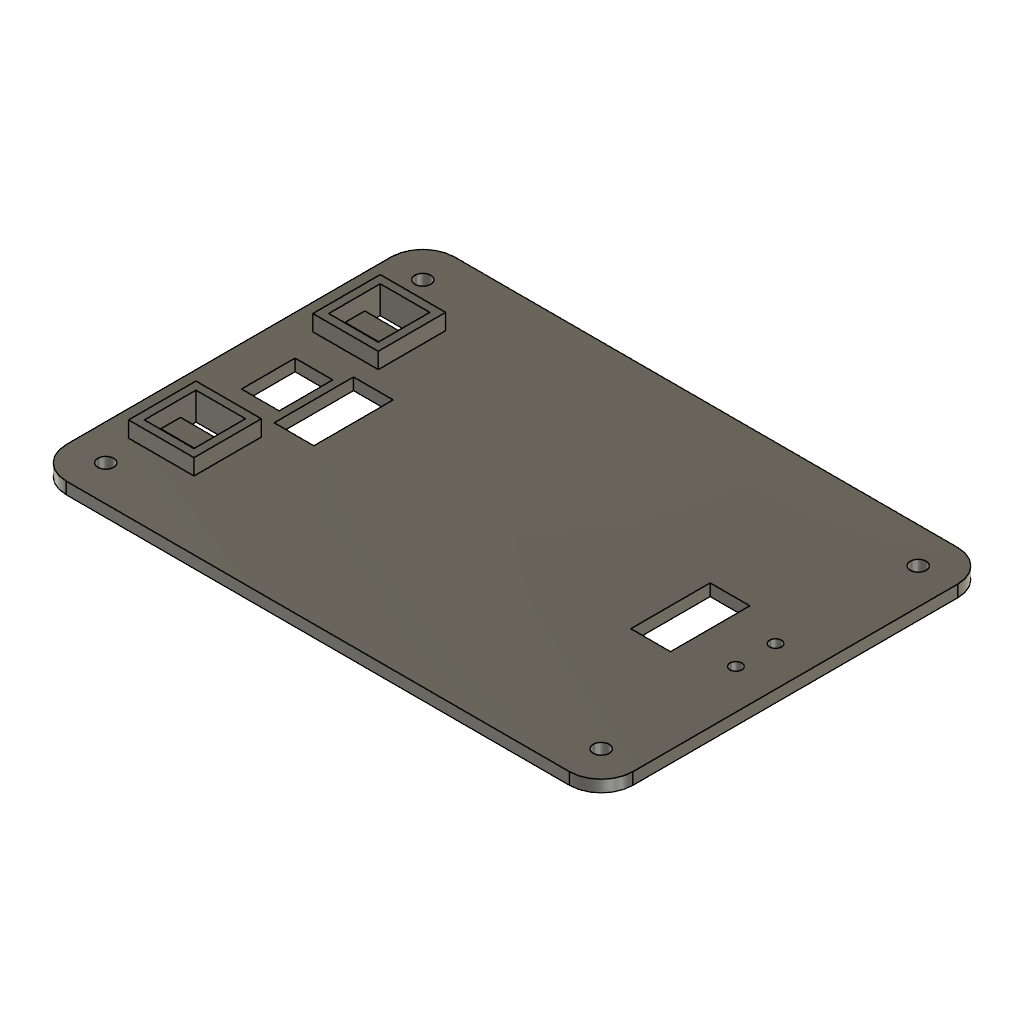
Tapa de la PCB (Autodesk Fusion 360 design; units mm, degrees)
Autodesk Fusion 360 part; units mm, degrees
sketch "Boceto1" plane through (0, 0, 0) normal (0, 0, 1) x (1, 0, 0)
  line L0 (71.5, 0) -> (-71.5, 0)
  line L1 (0, -49) -> (0, 49)
  line L2 (-71.5, 49) -> (71.5, 49)
  line L3 (71.5, 49) -> (71.5, -49)
  line L4 (71.5, -49) -> (-71.5, -49)
  line L5 (-71.5, -49) -> (-71.5, 49)
  line L6 (-71.5, 49) -> (71.5, -49) construction
  line L7 (71.5, 49) -> (-71.5, -49) construction
  dimension "d1" = 143
  dimension "d2" = 98
  constraint midpoint L0 origin
  constraint horizontal L0
  constraint midpoint L1 origin
  constraint perpendicular L0 L1
  constraint horizontal L2
  constraint perpendicular L2 L3
  constraint parallel L2 L4
  constraint parallel L3 L5
  constraint coincident L6 origin
  constraint coincident L7 origin
  measures "d1" distance of L0.start L0.end
  measures "d2" distance of L1.start L1.end
extrude "Extruir1" add sketch "Boceto1" along normal blind 3
sketch "Boceto2" plane through (0, 0, 3) normal (0, 0, 1) x (-1, 0, 0)
  line L0 (71.5, 49) -> (-71.5, 49)
  line L1 (-71.5, 49) -> (-71.5, -49)
  line L2 (-71.5, -49) -> (71.5, -49)
  line L3 (71.5, -49) -> (71.5, 49)
  line L4 (71.5, -49) -> (62.5, -49)
  line L5 (62.5, -49) -> (62.5, -40)
  line L6 (71.5, 49) -> (62.5, 49)
  line L7 (62.5, 49) -> (62.5, 40)
  line L8 (-71.5, 49) -> (-71.5, 40)
  line L9 (-71.5, 40) -> (-62.5, 40)
  line L10 (-71.5, -49) -> (-62.5, -49)
  line L11 (-62.5, -49) -> (-62.5, -40)
  circle A0 centre (62.5, -40) radius 2
  circle A1 centre (62.5, 40) radius 2
  circle A2 centre (-62.5, -40) radius 2
  circle A3 centre (-62.5, 40) radius 2
  dimension "d7" = 9
  dimension "d8" = 9
  dimension "d9" = 9
  dimension "d10" = 9
  dimension "d11" = 9
  dimension "d12" = 9
  dimension "d13" = 9
  dimension "d14" = 9
  dimension "d15" = 4
  dimension "d16" = 4
  dimension "d17" = 4
  dimension "d18" = 4
  constraint coincident L2.end L3.start
  constraint perpendicular L3 L4
  constraint perpendicular L2 L5
  constraint coincident L0.start L3.end
  constraint perpendicular L3 L6
  constraint perpendicular L6 L7
  constraint coincident L0.end L1.start
  constraint perpendicular L0 L8
  constraint perpendicular L1 L9
  constraint coincident L1.end L2.start
  constraint perpendicular L1 L10
  constraint perpendicular L2 L11
  constraint coincident L5.end A0.centre
  constraint coincident L7.end A1.centre
  constraint coincident L11.end A2.centre
  constraint coincident L9.end A3.centre
  measures "d7" distance of L2.end L4.end
  measures "d8" distance of L4.end L5.end
  measures "d9" distance of L0.start L6.end
  measures "d10" distance of L6.end L7.end
  measures "d11" distance of L0.end L8.end
  measures "d12" distance of L8.end L9.end
  measures "d13" distance of L1.end L10.end
  measures "d14" distance of L10.end L11.end
  measures "d15" diameter of A0
  measures "d16" diameter of A1
  measures "d17" diameter of A2
  measures "d18" diameter of A3
extrude "Extruir2" cut sketch "Boceto2" against normal blind 3 contours A0 | A1 | A2 | A3
fillet "Empalme2" radius 8 4 edges at (-71.5, -49, 1.5) (-71.5, 49, 1.5) (71.5, -49, 1.5) (71.5, 49, 1.5)
sketch "Boceto3" plane through (0, 0, 3) normal (0, 0, 1) x (-1, 0, 0)
  circle A0 centre (62.5, 40) radius 2
  circle A1 centre (-62.5, -40) radius 2
  circle A2 centre (62.5, -40) radius 2
  circle A3 centre (-62.5, 40) radius 2
  arc A4 (-71.5, -41) -> (-63.5, -49) centre (-63.5, -41) ccw
  line L0 (-63.5, -49) -> (63.5, -49)
  arc A5 (63.5, -49) -> (71.5, -41) centre (63.5, -41) ccw
  line L1 (71.5, -41) -> (71.5, 41)
  arc A6 (71.5, 41) -> (63.5, 49) centre (63.5, 41) ccw
  line L2 (63.5, 49) -> (-63.5, 49)
  arc A7 (-63.5, 49) -> (-71.5, 41) centre (-63.5, 41) ccw
  line L3 (-71.5, 41) -> (-71.5, -41)
  line L4 (-40, 0) -> (40, 0)
  line L5 (40, 10) -> (40, -10)
  line L6 (-40, 10) -> (-40, -10)
  line L7 (40, -10) -> (50, -10)
  line L8 (50, -10) -> (50, 10)
  line L9 (50, 10) -> (40, 10)
  line L10 (40, 10) -> (40, -10)
  line L11 (-40, -10) -> (-50, -10)
  line L12 (-50, -10) -> (-50, 10)
  line L13 (-50, 10) -> (-40, 10)
  line L14 (-40, 10) -> (-40, -10)
  dimension "d23" = 80
  dimension "d24" = 20
  dimension "d25" = 20
  dimension "d26" = 10
  dimension "d27" = 20
  dimension "d28" = 10
  dimension "d29" = 20
  constraint midpoint L4 origin
  constraint horizontal L4
  constraint midpoint L4.end L5
  constraint perpendicular L4 L5
  constraint midpoint L4.start L6
  constraint perpendicular L4 L6
  constraint horizontal L7
  constraint vertical L8
  constraint horizontal L9
  constraint vertical L10
  constraint horizontal L11
  constraint vertical L12
  constraint horizontal L13
  constraint vertical L14
  measures "d23" distance of L4.start L4.end
  measures "d24" distance of L5.start L5.end
  measures "d25" distance of L6.start L6.end
  measures "d26" distance of L5.end L7.end
  measures "d27" distance of L5.end L5.start
  measures "d28" distance of L6.end L11.end
  measures "d29" distance of L6.end L6.start
extrude "Extruir3" cut sketch "Boceto3" against normal blind 3 contours L5 L7 L8 L9 L10 | L6 L11 L12 L13 L14
sketch "Boceto4" plane through (0, 0, 3) normal (0, 0, 1) x (-1, 0, 0)
  line L0 (50, -10) -> (40, -10)
  line L1 (40, -10) -> (40, 10)
  line L2 (40, 10) -> (50, 10)
  line L3 (50, 10) -> (50, -10)
  line L4 (-50, -10) -> (-50, 10)
  line L5 (-50, 10) -> (-40, 10)
  line L6 (-40, 10) -> (-40, -10)
  line L7 (-40, -10) -> (-50, -10)
  circle A0 centre (62.5, 40) radius 2
  circle A1 centre (-62.5, -40) radius 2
  circle A2 centre (62.5, -40) radius 2
  circle A3 centre (-62.5, 40) radius 2
  arc A4 (-71.5, -41) -> (-63.5, -49) centre (-63.5, -41) ccw
  line L8 (-63.5, -49) -> (63.5, -49)
  arc A5 (63.5, -49) -> (71.5, -41) centre (63.5, -41) ccw
  line L9 (71.5, -41) -> (71.5, 41)
  arc A6 (71.5, 41) -> (63.5, 49) centre (63.5, 41) ccw
  line L10 (63.5, 49) -> (-63.5, 49)
  arc A7 (-63.5, 49) -> (-71.5, 41) centre (-63.5, 41) ccw
  line L11 (-71.5, 41) -> (-71.5, -41)
  line L12 (71.5, 0) -> (61.5, 0)
  line L13 (61.5, 6.75) -> (61.5, -6.75)
  line L14 (61.5, -6.75) -> (52, -6.75)
  line L15 (61.5, 6.75) -> (52, 6.75)
  line L16 (52, 6.75) -> (52, -6.75)
  dimension "d32" = 10
  dimension "d33" = 13.5
  dimension "d34" = 9.5
  dimension "d35" = 9.5
  constraint midpoint L9 L12.start
  constraint perpendicular L9 L12
  constraint midpoint L12.end L13
  constraint perpendicular L12 L13
  constraint perpendicular L13 L14
  constraint perpendicular L13 L15
  measures "d32" distance of L12.start L12.end
  measures "d33" distance of L13.start L13.end
  measures "d34" distance of L13.end L14.end
  measures "d35" distance of L13.start L15.end
extrude "Extruir4" cut sketch "Boceto4" against normal blind 3 contours L13 L14 L15 L16
sketch "Boceto5" plane through (0, 0, 3) normal (0, 0, 1) x (-1, 0, 0)
  line L0 (52, -6.75) -> (52, 6.75)
  line L1 (52, 6.75) -> (61.5, 6.75)
  line L2 (61.5, 6.75) -> (61.5, -6.75)
  line L3 (61.5, -6.75) -> (52, -6.75)
  line L4 (50, -10) -> (40, -10)
  line L5 (40, -10) -> (40, 10)
  line L6 (40, 10) -> (50, 10)
  line L7 (50, 10) -> (50, -10)
  line L8 (-50, -10) -> (-50, 10)
  line L9 (-50, 10) -> (-40, 10)
  line L10 (-40, 10) -> (-40, -10)
  line L11 (-40, -10) -> (-50, -10)
  circle A0 centre (62.5, 40) radius 2
  circle A1 centre (-62.5, -40) radius 2
  circle A2 centre (62.5, -40) radius 2
  circle A3 centre (-62.5, 40) radius 2
  arc A4 (-71.5, -41) -> (-63.5, -49) centre (-63.5, -41) ccw
  line L12 (-63.5, -49) -> (63.5, -49)
  arc A5 (63.5, -49) -> (71.5, -41) centre (63.5, -41) ccw
  line L13 (71.5, -41) -> (71.5, 41)
  arc A6 (71.5, 41) -> (63.5, 49) centre (63.5, 41) ccw
  line L14 (63.5, 49) -> (-63.5, 49)
  arc A7 (-63.5, 49) -> (-71.5, 41) centre (-63.5, 41) ccw
  line L15 (-71.5, 41) -> (-71.5, -41)
  line L16 (56.75, 6.75) -> (56.75, 16.75)
  line L17 (56.75, -6.75) -> (56.75, -16.75)
  line L18 (63, 16.75) -> (50.5, 16.75)
  line L19 (63, -16.75) -> (50.5, -16.75)
  line L20 (50.5, 16.75) -> (50.5, 29.75)
  line L21 (50.5, -16.75) -> (50.5, -29.75)
  line L22 (50.5, -29.75) -> (63, -29.75)
  line L23 (63, -29.75) -> (63, -16.75)
  line L24 (50.5, 29.75) -> (63, 29.75)
  line L25 (63, 29.75) -> (63, 16.75)
  line L26 (50.5, 25.6389) -> (50.5, 20.6389)
  line L27 (50.5, -20.8611) -> (50.5, -25.8611)
  line L28 (50.5, -25.8611) -> (63, -25.8611)
  line L29 (50.5, -20.8611) -> (63, -20.8611)
  line L30 (50.5, 20.6389) -> (63, 20.6389)
  line L31 (50.5, 25.6389) -> (63, 25.6389)
  line L32 (65, -31.75) -> (65, -14.75)
  line L33 (65, -14.75) -> (48.5, -14.75)
  line L34 (48.5, -14.75) -> (48.5, -31.75)
  line L35 (48.5, -31.75) -> (65, -31.75)
  line L36 (65, 31.75) -> (65, 14.75)
  line L37 (65, 14.75) -> (48.5, 14.75)
  line L38 (48.5, 14.75) -> (48.5, 31.75)
  line L39 (48.5, 31.75) -> (65, 31.75)
  point P0 (50.5, 23.1389)
  point P1 (50.5, -23.3611)
  dimension "d38" = 10
  dimension "d39" = 10
  dimension "d40" = 12.5
  dimension "d41" = 12.5
  dimension "d42" = 13
  dimension "d43" = 13
  dimension "d44" = 12.5
  dimension "d45" = 12.5
  dimension "d46" = 5
  dimension "d47" = 5
  dimension "d48" = 2
  dimension "d49" = -2
  constraint midpoint L1 L16.start
  constraint perpendicular L1 L16
  constraint midpoint L3 L17.start
  constraint perpendicular L3 L17
  constraint midpoint L16.end L18
  constraint perpendicular L16 L18
  constraint midpoint L17.end L19
  constraint perpendicular L17 L19
  constraint perpendicular L18 L20
  constraint perpendicular L19 L21
  constraint perpendicular L21 L22
  constraint perpendicular L20 L24
  constraint midpoint L26 P0
  constraint coincident L20 P0
  constraint perpendicular L24 L26
  constraint midpoint L27 P1
  constraint coincident L21 P1
  constraint perpendicular L3 L27
  constraint coincident L23 L28.end
  constraint perpendicular L23 L28
  constraint coincident L23 L29.end
  constraint perpendicular L23 L29
  constraint coincident L25 L30.end
  constraint perpendicular L25 L30
  constraint coincident L25 L31.end
  constraint perpendicular L25 L31
  measures "d38" distance of L16.start L16.end
  measures "d39" distance of L17.start L17.end
  measures "d40" distance of L18.start L18.end
  measures "d41" distance of L19.start L19.end
  measures "d42" distance of L18.end L20.end
  measures "d43" distance of L19.end L21.end
  measures "d44" distance of L21.end L22.end
  measures "d45" distance of L20.end L24.end
  measures "d46" distance of L26.start L26.end
  measures "d47" distance of L27.start L27.end
extrude "Extruir5" add sketch "Boceto5" along normal blind 4 contours L32 L33 L34 L35 | L36 L37 L38 L39
extrude "Extruir6" cut sketch "Boceto5" against normal blind 3 contours L18 L20 L25 L30 | L20 L24 L25 L31 | L19 L21 L23 L29 | L21 L22 L23 L28
sketch "Boceto6" plane through (0, 0, 3) normal (0, 0, 1) x (-1, 0, 0)
  line L0 (48.5, -31.75) -> (48.5, -14.75)
  line L1 (48.5, -14.75) -> (65, -14.75)
  line L2 (65, -14.75) -> (65, -31.75)
  line L3 (65, -31.75) -> (48.5, -31.75)
  line L4 (52, -6.75) -> (52, 6.75)
  line L5 (52, 6.75) -> (61.5, 6.75)
  line L6 (61.5, 6.75) -> (61.5, -6.75)
  line L7 (61.5, -6.75) -> (52, -6.75)
  line L8 (50, -10) -> (40, -10)
  line L9 (40, -10) -> (40, 10)
  line L10 (40, 10) -> (50, 10)
  line L11 (50, 10) -> (50, -10)
  line L12 (-50, -10) -> (-50, 10)
  line L13 (-50, 10) -> (-40, 10)
  line L14 (-40, 10) -> (-40, -10)
  line L15 (-40, -10) -> (-50, -10)
  circle A0 centre (62.5, 40) radius 2
  circle A1 centre (-62.5, -40) radius 2
  circle A2 centre (62.5, -40) radius 2
  circle A3 centre (-62.5, 40) radius 2
  arc A4 (-71.5, -41) -> (-63.5, -49) centre (-63.5, -41) ccw
  line L16 (-63.5, -49) -> (63.5, -49)
  arc A5 (63.5, -49) -> (71.5, -41) centre (63.5, -41) ccw
  line L17 (71.5, -41) -> (71.5, 41)
  arc A6 (71.5, 41) -> (63.5, 49) centre (63.5, 41) ccw
  line L18 (63.5, 49) -> (-63.5, 49)
  arc A7 (-63.5, 49) -> (-71.5, 41) centre (-63.5, 41) ccw
  line L19 (-71.5, 41) -> (-71.5, -41)
  line L20 (48.5, 31.75) -> (65, 31.75)
  line L21 (65, 31.75) -> (65, 14.75)
  line L22 (65, 14.75) -> (48.5, 14.75)
  line L23 (48.5, 14.75) -> (48.5, 31.75)
  line L24 (-71.5, 0) -> (-61.5, 0)
  line L25 (-61.5, -5) -> (-61.5, 5)
  circle A8 centre (-61.5, 5) radius 1.5
  circle A9 centre (-61.5, -5) radius 1.5
  dimension "d54" = 10
  dimension "d55" = 10
  dimension "d56" = 3
  dimension "d57" = 3
  constraint midpoint L19 L24.start
  constraint perpendicular L19 L24
  constraint midpoint L24.end L25
  constraint perpendicular L24 L25
  constraint coincident L25.end A8.centre
  constraint coincident L25.start A9.centre
  measures "d54" distance of L24.start L24.end
  measures "d55" distance of L25.start L25.end
  measures "d56" diameter of A8
  measures "d57" diameter of A9
extrude "Extruir7" cut sketch "Boceto6" against normal blind 3 contours A8 | A9
